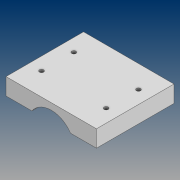
# Autodesk Inventor part: 19_Kep_han_B
Saved by Autodesk Inventor 2021 (Build 250183000, 183)
## iProperties
Created: 2024-04-05
Part Number: 19_Kep_han_B
Material: Generic
Document SubType Name: Modeling
Designer: Admin
Density: 1 g/cm^3
Appearance: Default
Author: Admin
Autodesk Inventor part; units mm, degrees
ref_plane "YZ Plane" through (0, 0, 0) normal (1, 0, 0) x (0, 1, 0)
ref_plane "XZ Plane" through (0, 0, 0) normal (0, 1, 0) x (-1, 0, 0)
ref_plane "XY Plane" through (0, 0, 0) normal (0, 0, 1) x (1, 0, 0)
sketch "Sketch1" plane through (0, 0, 0) normal (0, 0, 1) x (1, 0, 0)
  line L0 (-35, -6.5) -> (35, -6.5)
  line L1 (35, -6.5) -> (35, 6.5)
  line L2 (35, 6.5) -> (-35, 6.5)
  line L3 (-35, 6.5) -> (-35, -6.5)
  line L4 (-35, -6.5) -> (35, 6.5) construction
  line L5 (35, -6.5) -> (-35, 6.5) construction
  circle A0 centre (0, -16.5) radius 18
  line L6 (0, 6.5) -> (0, -6.5) construction
  point P0 (0, 0)
  point P1 (0, 0)
  point P2 (-14.9666, -6.5)
  point P3 (14.9666, -6.5)
  dimension "d0" = 36
  dimension "d1" = 10
  dimension "d2" = 70
  dimension "d3" = 13
  constraints: 14 end point, 5 midpoint, 2 parallel, 1 centre point, 1 horizontal, 1 perpendicular, 1 vertical alignment
  measures "d0" diameter of A0
  measures "d1" distance from line of L0 A0.centre
  measures "d2" distance between parallel lines of L3 L1
  measures "d3" distance between parallel lines of L0 L2
extrude "Extrusion1" add sketch "Sketch1" along normal mid plane 60 contours L3 L2 L1 L0 A0
sketch "Sketch2" plane through (14.9666, -6.5, -30) normal (0, -1, 0) x (1, 0, 0)
  line L0 (-29.9333, 0) -> (-49.9666, 0) projected
  line L1 (-29.9333, 0) -> (-29.9333, 60) projected
  line L2 (-49.9666, 60) -> (-29.9333, 60) projected
  line L3 (-49.9666, 60) -> (-49.9666, 0) projected
  line L4 (20.0334, 0) -> (0, 0) projected
  line L5 (20.0334, 0) -> (20.0334, 60) projected
  line L6 (0, 60) -> (20.0334, 60) projected
  line L7 (0, 0) -> (0, 60) projected
  line L8 (-49.9666, 60) -> (-29.9333, 60) projected
  line L9 (-39.9499, 60) -> (-39.9499, 0)
  line L10 (-29.9333, 0) -> (-49.9666, 0) projected
  line L11 (20.0334, 0) -> (0, 0) projected
  line L12 (10.0167, 0) -> (10.0167, 60)
  line L13 (-49.9666, 30) -> (20.0334, 30) construction
  line L14 (-49.9666, 17.5) -> (20.0334, 17.5)
  line L15 (20.0334, 17.5) -> (20.0334, 42.5)
  line L16 (20.0334, 42.5) -> (-49.9666, 42.5)
  line L17 (-49.9666, 42.5) -> (-49.9666, 17.5)
  line L18 (-49.9666, 17.5) -> (20.0334, 42.5) construction
  line L19 (20.0334, 17.5) -> (-49.9666, 42.5) construction
  point P0 (-14.9666, 30)
  point P1 (-39.9499, 42.5)
  point P2 (-39.9499, 17.5)
  point P3 (10.0167, 17.5)
  point P4 (10.0167, 42.5)
  dimension "d6" = 25
  constraints: 18 end point, 9 midpoint, 9 point on line, 2 parallel, 1 horizontal, 1 perpendicular
  measures "d6" distance between parallel lines of L14 L16
hole "Hole1" at (-24.9833, -6.5, 12.5) at (-24.9833, -6.5, -12.5) at (24.9833, -6.5, -12.5) at (24.9833, -6.5, 12.5) direction (0, 1, 0) diameter 3.2 end through all
body "Solid1"
